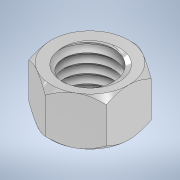
# Autodesk Inventor part: Nut
Saved by Autodesk Inventor 2022 (Build 260153000, 153)
## iProperties
Created: 2021-08-27
Part Number: Nut
Material: Aluminum 6061-AHC
Document SubType Name: Modeling
Designer: ancem
Density: 2.7 g/cm^3
Appearance: Aluminum - Dark
Author: ancem
Autodesk Inventor part; units mm, degrees
ref_plane "YZ Plane" through (0, 0, 0) normal (1, 0, 0) x (0, 1, 0)
ref_plane "XZ Plane" through (0, 0, 0) normal (0, 1, 0) x (-1, 0, 0)
ref_plane "XY Plane" through (0, 0, 0) normal (0, 0, 1) x (1, 0, 0)
sketch "Sketch1" plane through (0, 0, 0) normal (0, 1, 0) x (-1, 0, 0)
  line L0 (-6.5, -3.7528) -> (-6.5, 3.7528)
  line L1 (-6.5, 3.7528) -> (0, 7.5056)
  line L2 (0, 7.5056) -> (6.5, 3.7528)
  line L3 (6.5, 3.7528) -> (6.5, -3.7528)
  line L4 (6.5, -3.7528) -> (0, -7.5056)
  line L5 (0, -7.5056) -> (-6.5, -3.7528)
  point P0 (0, 0)
  point P1 (0, 0)
  dimension "d0" = 13
  constraints: 12 end point, 1 coincident, 1 vertical, 13 other
  measures "d0" distance between parallel lines of L5 L2
extrude "Extrusion1" add sketch "Sketch1" along normal mid plane 8
sketch "Sketch2" plane through (0, 4, 0) normal (0, 1, 0) x (1, 0, 0)
  circle A0 centre (0, 0) radius 6.5
  line L0 (6.5, 3.7528) -> (0, 7.5056) projected
  constraints: 1 centre point, 1 coincident, 1 tangent
extrude "Extrusion2" cut sketch "Sketch2" against normal through all draft 45 keep common part
sketch "Sketch3" plane through (0, -4, 0) normal (0, -1, 0) x (1, 0, 0)
  circle A0 centre (0, 0) radius 6.5
  line L0 (-6.5, -3.7528) -> (0, -7.5056) projected
  constraints: 1 centre point, 1 coincident, 1 tangent
extrude "Extrusion3" cut sketch "Sketch3" against normal through all draft 45 keep common part
sketch "Sketch4" plane through (0, -4, 0) normal (0, -1, 0) x (1, 0, 0)
  circle A0 centre (0, 0) radius 4
  dimension "d7" = 8
  constraints: 1 centre point, 1 coincident
  measures "d7" diameter of A0
extrude "Extrusion4" cut sketch "Sketch4" against normal blind 10
chamfer "Chamfer1" distance 0.5 angle 45 2 edges at (-4, -4, 0) (-4, 4, 0)
sketch "Sketch5" plane through (0, 0, 0) normal (0, 0, 1) x (1, 0, 0)
  line L0 (4, -13.2069) -> (4, -11.5069)
  line L1 (4, -11.5069) -> (5.1722, -12.1837)
  line L2 (5.1722, -12.5301) -> (4, -13.2069)
  line L3 (4, -12.3569) -> (5.4722, -12.3569)
  arc A0 (5.1722, -12.5301) -> (5.1722, -12.1837) centre (5.0722, -12.3569) ccw
  line L4 (0, 2.9944) -> (0, -2.9944) projected
  point P0 (0, 0)
  dimension "d13" = 1.7
  dimension "d14" = 60
  dimension "d15" = 0.2
  dimension "d16" = 4
  constraints: 8 end point, 2 point on circle, 2 point on line, 2 tangent, 1 centre point, 1 horizontal, 1 midpoint, 1 vertical
  measures "d13" distance of L0.start L0.end
  measures "d14" angle of L1 L2
  measures "d15" radius of A0
  measures "d16" distance between parallel lines of L4 L0
coil "Coil1" sketch "Sketch5" operation cut axis through (0, -10, 0) along (0, 1, 0) pitch 1.5 turns 13.333333 hand right
body "Solid1"
